Mast 1 (Autodesk Fusion 360 design; units mm, degrees)
Autodesk Fusion 360 part; units mm, degrees
sketch "Sketch3" plane through (0, 0, 0) normal (0, 0, 1) x (-1, 0, 0)
  circle A0 centre (13, -13) radius 1
  circle A1 centre (13, 13) radius 1
  circle A2 centre (-13, 13) radius 1
  circle A3 centre (-13, -13) radius 1
  circle A4 centre (13, -13) radius 1.6
  circle A5 centre (13, 13) radius 1.6
  circle A6 centre (-13, 13) radius 1.6
  circle A7 centre (-13, -13) radius 1.6
  line L0 (17.5, -14.8) -> (17.5, 14.8)
  line L1 (17.5, 14.8) -> (15.3, 17)
  line L2 (15.3, 17) -> (-15.3, 17)
  line L3 (-15.3, 17) -> (-17.5, 14.8)
  line L4 (-17.5, 14.8) -> (-17.5, -14.8)
  line L5 (-17.5, -14.8) -> (-15.3, -17)
  line L6 (-15.3, -17) -> (15.3, -17)
  line L7 (15.3, -17) -> (17.5, -14.8)
  circle A8 centre (0, 0) radius 11.65
  circle A9 centre (0, 0) radius 8.65
  line L8 (8.5, 17) -> (-8.5, 17)
  line L9 (-8.5, 17) -> (-8.5, 12)
  line L10 (-8.5, 12) -> (8.5, 12)
  line L11 (8.5, 12) -> (8.5, 17)
  line L12 (8.5, -17) -> (-8.5, -17)
  line L13 (-8.5, -17) -> (-8.5, -12)
  line L14 (-8.5, -12) -> (8.5, -12)
  line L15 (8.5, -12) -> (8.5, -17)
  point P0 (17.5, -14.8)
  point P1 (15.3, -17)
  point P2 (17.5, 14.8)
  point P3 (15.3, 17)
  point P4 (-15.3, 17)
  point P5 (-17.5, 14.8)
  point P6 (-17.5, -14.8)
  point P7 (-15.3, -17)
  point P8 (-17.5, -8.8262)
  point P9 (-17.5, 8.8262)
  point P10 (-9, 17)
  point P11 (9, 17)
  point P12 (9, -17)
  point P13 (-9, -17)
  dimension "d26" = 3.2
  dimension "d27" = 3.2
  dimension "d28" = 3.2
  dimension "d29" = 3.2
  dimension "d30" = 23.3
  dimension "d31" = -3
  dimension "d38" = 5
  dimension "d39" = 0.5
  dimension "d40" = 0.5
  dimension "d41" = 0.5
  dimension "d42" = 5
  dimension "d43" = 0.5
  constraint concentric A0 A4
  constraint concentric A1 A5
  constraint concentric A2 A6
  constraint concentric A3 A7
  constraint coincident P0 L0.start
  constraint coincident P2 L0.end
  constraint coincident P3 L1.end
  constraint coincident P4 L2.end
  constraint coincident P5 L3.end
  constraint coincident P6 L4.end
  constraint coincident P7 L5.end
  constraint coincident P1 L6.end
  constraint coincident A8.centre A9.centre
  constraint horizontal L8
  constraint vertical L9
  constraint horizontal L10
  constraint vertical L11
  constraint coincident L2 L8.start
  constraint horizontal L12
  constraint vertical L13
  constraint horizontal L14
  constraint vertical L15
  constraint coincident L6 L12.start
  measures "d26" diameter of A4
  measures "d27" diameter of A5
  measures "d28" diameter of A6
  measures "d29" diameter of A7
  measures "d30" diameter of A8
  measures "d38" distance of L8.start L10.end
  measures "d39" distance of P11 L8.start
  measures "d40" distance of P10 L8.end
  measures "d41" distance of P12 L12.start
  measures "d42" distance of L12.start L14.end
  measures "d43" distance of P13 L12.end
extrude "Extrude6" add sketch "Sketch3" against normal blind 3 contours L6 L12 L13 L14 L15 | L2 L8 L9 L10 L11 makes body 1 at (2.8333, -15.3333, 0) makes body 2 at (-2.8333, 13.6667, 0)
extrude "Extrude3" add sketch "Sketch3" along normal blind 3 contours L0 L1 L2 L3 L4 L5 L6 L7 L9 L10 L11 L13 L14 L15 | L6 L12 L13 L14 L15 | L2 L8 L9 L10 L11 | A8 bodies 1 2
extrude "Extrude4" cut sketch "Sketch3" along normal blind 40 contours A8 bodies 1
extrude "Extrude5" add sketch "Sketch3" along normal blind 50 contours A8 bodies 1
sketch "Sketch4" plane through (17.5, 0, 0) normal (1, 0, 0) x (0, 1, 0)
  line L0 (-14.8, 0) -> (14.8, 0)
  line L1 (14.8, 0) -> (14.8, 3)
  line L2 (14.8, 3) -> (-14.8, 3)
  line L3 (-14.8, 3) -> (-14.8, 0)
  line L4 (1.289, 2.5498) -> (9.3, 0)
  line L5 (-1.289, 2.5498) -> (-9.3, 0)
  arc A0 (1.289, 2.5498) -> (-1.289, 2.5498) centre (0, -1.5) ccw
  line L6 (0, 0) -> (0, -1.5) construction
  dimension "d50" = 4.25
  dimension "d51" = 5.5
  dimension "d52" = 5.5
  dimension "d54" = 1.5
  constraint coincident L0 L4.end
  constraint coincident L0 L5.end
  constraint coincident L6.start origin
  constraint perpendicular L0 L6
  constraint coincident A0.centre L6.end
  constraint tangent L4 A0
  constraint tangent L5 A0
  measures "d50" radius of A0
  measures "d51" distance of L0.end L4.end
  measures "d52" distance of L0.start L5.end
  measures "d54" distance of L6.start A0.centre
extrude "Extrude7" cut sketch "Sketch4" against normal through all contours L0 L4 L5 A0 bodies 1
